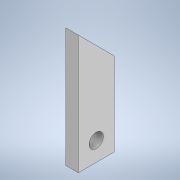
# Autodesk Inventor part: locker
Saved by Autodesk Inventor 2021 (Build 250183000, 183)
## iProperties
Created: 2020-06-28
Part Number: locker
Material: Generic
Document SubType Name: Modeling
Designer: Yatekii
Density: 1 g/cm^3
Appearance: Default
Author: Yatekii
Autodesk Inventor part; units mm, degrees
ref_plane "YZ Plane" through (0, 0, 0) normal (1, 0, 0) x (0, 1, 0)
ref_plane "XZ Plane" through (0, 0, 0) normal (0, 1, 0) x (-1, 0, 0)
ref_plane "XY Plane" through (0, 0, 0) normal (0, 0, 1) x (1, 0, 0)
sketch "Sketch1" plane through (0, 0, 0) normal (0, 1, 0) x (-1, 0, 0)
  line L0 (-1.3, -3.75) -> (1.3, -3.75)
  line L1 (1.3, -3.75) -> (1.3, 3.75)
  line L2 (1.3, 3.75) -> (-1.3, 3.75)
  line L3 (-1.3, 3.75) -> (-1.3, -3.75)
  line L4 (-1.3, -3.75) -> (1.3, 3.75) construction
  line L5 (1.3, -3.75) -> (-1.3, 3.75) construction
  point P0 (0, 0)
  dimension "d0" = 2.6
  dimension "d1" = 7.5
  constraints: 12 end point, 2 midpoint, 2 parallel, 1 horizontal, 1 perpendicular
  measures "d0" distance of L2.end L1.end
  measures "d1" distance of L1.end L0.end
extrude "Extrusion1" add sketch "Sketch1" along normal blind 25
chamfer "Chamfer1" distance 7.5 angle 45 1 edges at (0, 25, -3.75)
sketch "Sketch2" plane through (1.3, 0, 3.75) normal (1, 0, 0) x (0, 0, -1)
  circle A0 centre (3.75, 4) radius 1.5
  point P0 (3.75, 0)
  dimension "d7" = 3
  dimension "d8" = 4
  constraints: 1 centre point
  measures "d7" diameter of A0
  measures "d8" distance of point (3.75, 0) A0.centre
extrude "Extrusion2" cut sketch "Sketch2" against normal blind 16
body "Solid1"
